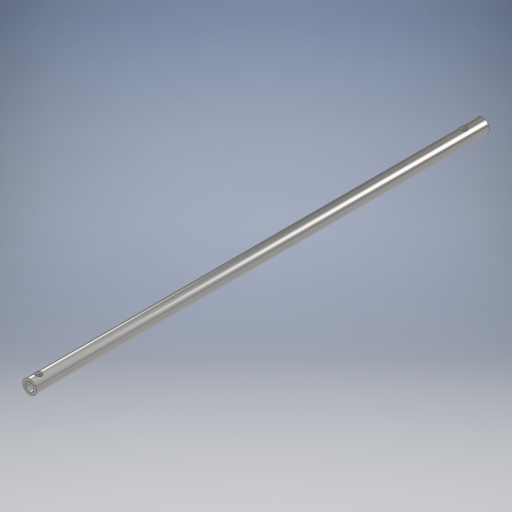
# Autodesk Inventor part: driveshaft
Saved by Autodesk Inventor 2024 (Build 280153000, 153)
## iProperties
Created: 2024-04-13
Part Number: driveshaft
Material: Steel, Mild
Document SubType Name: Modeling
Designer: Alex
Density: 7.85 g/cm^3
Appearance: Semi-Polished
Author: Alex
Autodesk Inventor part; units mm, degrees
ref_plane "YZ Plane" through (0, 0, 0) normal (1, 0, 0) x (0, 1, 0)
ref_plane "XY Plane" through (0, 0, 0) normal (0, 0, 1) x (1, 0, 0)
sketch "Sketch1" plane through (0, 0, 0) normal (0, 0, 1) x (1, 0, 0)
  circle A0 centre (0, 0) radius 4
  dimension "d0" = 8
  constraints: 1 centre point, 1 coincident
  measures "d0" diameter of A0
extrude "Extrusion1" add sketch "Sketch1" against normal blind 260
ref_plane "Work Plane1" through (0, 4, 0) normal (0, 1, 0) x (-1, 0, 0)
sketch "Sketch2" plane through (0, 4, 0) normal (0, 1, 0) x (-1, 0, 0)
  line L0 (-4, -260) -> (4, -260) construction
  line L1 (4, 0) -> (-4, 0) construction
  point P0 (0, 0)
  point P1 (0, -5)
  dimension "d11" = 5
  measures "d11" distance from line of L1 point (0, -5)
hole "Hole1" at (0, 4, -5) direction (0, -1, 0) diameter 3.688 end through all
sketch "Sketch3" plane through (0, 4, 0) normal (0, 1, 0) x (-1, 0, 0)
  line L0 (-4, -260) -> (4, -260) construction
  line L1 (0, -260) -> (0, -249.076) construction
  point P0 (0, 0)
  dimension "d12" = 10.924
  constraints: 2 end point, 1 coincident, 1 midpoint, 1 vertical
  measures "d12" distance of L1.start L1.end
hole "Hole2" at (0, 4, -249.076) direction (0, -1, 0) diameter 3.688 end through all
sketch "Sketch4" plane through (0, 0, 0) normal (0, 0, 1) x (1, 0, 0)
  circle A0 centre (0, 0) radius 2.5
  dimension "d20" = 5
  constraints: 1 centre point, 1 coincident
  measures "d20" diameter of A0
extrude "Extrusion2" cut sketch "Sketch4" against normal blind 13.274
body "Solid1"
